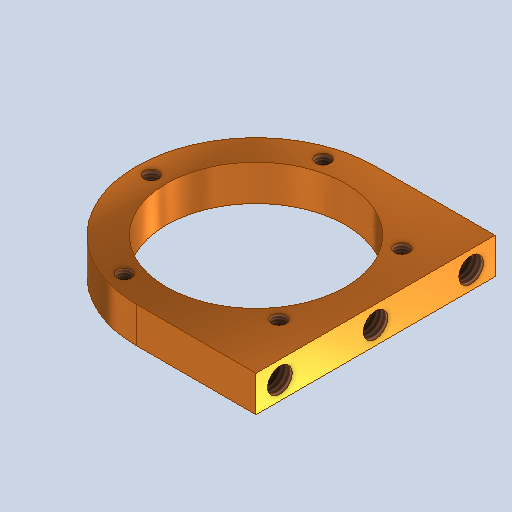
# Autodesk Inventor part: 34
Saved by Autodesk Inventor 2025.1 (Build 291241000, 241)
## iProperties
Created: 2024-09-17
Part Number: 34
Material: Gold
Document SubType Name: Modeling
Designer: ffogue
Density: 19.3 g/cm^3
Appearance: Metal 1600F Hot
Author: ffogue
Autodesk Inventor part; units mm, degrees
note: some values were not read from the file. Chosen so that the rebuilt part matches the saved one: direction of "Hole1".
ref_plane "YZ Plane" through (0, 0, 0) normal (1, 0, 0) x (0, 1, 0)
ref_plane "XZ Plane" through (0, 0, 0) normal (0, 1, 0) x (-1, 0, 0)
ref_plane "XY Plane" through (0, 0, 0) normal (0, 0, 1) x (1, 0, 0)
sketch "Sketch1" plane through (0, 0, 0) normal (0, 0, 1) x (1, 0, 0)
  line L0 (0, 20) -> (0, -20)
  line L1 (0, 20) -> (-20, 20)
  arc A0 (-20, 20) -> (-20, -20) centre (-20, 0) ccw
  line L2 (-20, -20) -> (0, -20)
  point P0 (0, 0)
  point P1 (0, 0)
  dimension "d0" = 20
  dimension "d1" = 20
  constraints: 6 end point, 2 point on circle, 1 centre point, 1 coincident, 1 horizontal, 1 horizontal alignment, 1 midpoint, 1 parallel, 1 tangent, 1 vertical
  measures "d0" distance of L0.start L1.end
  measures "d1" radius of A0
extrude "Extrusion1" add sketch "Sketch1" along normal blind 6
sketch "Sketch2" plane through (0, 0, 6) normal (0, 0, 1) x (1, 0, 0)
  circle A0 centre (-20, 0) radius 17.5 construction
  line L0 (0, -20) -> (0, 20) projected
  point P0 (0, 0)
  point P1 (0, 0)
  point P2 (-37.5, 0)
  point P3 (0, 0)
  dimension "d5" = 35
  dimension "d4" = 20
  constraints: 2 horizontal alignment, 2 midpoint, 2 other
  measures "d4" distance of point (0, 0) point (-20, 0)
hole "Hole1" at (-37.5, 0, 6) direction (0, 0, -1) diameter 2.459 depth 6 thread size "M3x0.5" class "6H" standard "ISO Metric profile"
pattern_circular "Circular Pattern1" count 5 over 360 about axis through (-20, 0, 0) along (0, 0, 1) of "Hole1"
sketch "Sketch4" plane through (0, -20, 0) normal (1, 0, 0) x (0, 0, -1)
  line L0 (0, 0) -> (0, 40) projected
  line L1 (0, 40) -> (-6, 40) projected
  point P0 (0, 20)
  point P1 (-3, 36)
  point P2 (-3, 20)
  point P3 (-3, 4)
  point P4 (0, 20)
  point P5 (-3, 40)
  dimension "d16" = 32
  dimension "d17" = 16
  constraints: 3 vertical alignment, 2 midpoint, 1 horizontal alignment
  measures "d16" distance of point (-3, 4) point (-3, 36)
  measures "d17" distance of point (-3, 20) point (-3, 36)
hole "Hole2" at (0, 16, 3) at (0, -16, 3) direction (-1, 0, 0) diameter 4.134 depth 14.2 thread size "M5x0.8" class "6H" standard "ISO Metric profile"
hole "Hole3" at (0, 0, 3) direction (-1, 0, 0) diameter 4.134 depth 14.2 thread size "M5x0.8" class "6H" standard "ISO Metric profile"
sketch "Sketch5" plane through (0, 0, 6) normal (0, 0, 1) x (1, 0, 0)
  circle A0 centre (-20, 0) radius 15
  line L0 (0, -20) -> (0, 20) projected
  arc A1 (-20, 20) -> (-20, -20) centre (-20, 0) ccw projected
  point P0 (0, 0)
  point P1 (0, 0)
  point P2 (0, 0)
  dimension "d32" = 30
  constraints: 2 horizontal alignment, 2 midpoint, 1 centre point, 1 concentric
  measures "d32" diameter of A0
extrude "Extrusion2" cut sketch "Sketch5" against normal up to surface (6 mm away)
equation "\"d17\" = 0.5 * d16"
body "Solid1"
